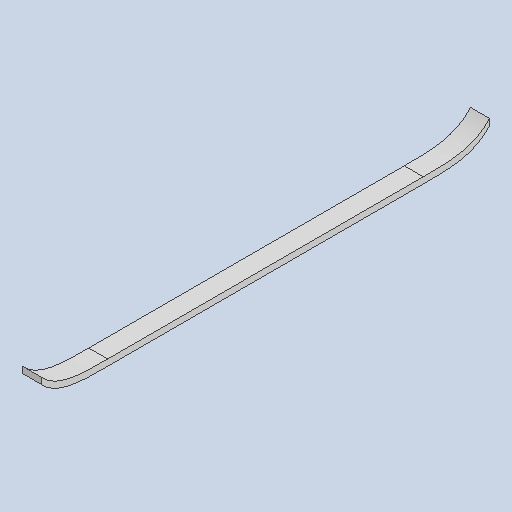
# Autodesk Inventor part: Landing_Skid
Saved by Autodesk Inventor 2027.1 (Build 311270010, 270A)
## iProperties
Created: 2026-09-09
Part Number: Landing_Skid
Material: Generic
Document SubType Name: Modeling
Designer: PWYNNE
Density: 1 g/cm^3
Appearance: Default
Author: PWYNNE
Autodesk Inventor part; units mm, degrees
ref_plane "YZ Plane" through (0, 0, 0) normal (1, 0, 0) x (0, 1, 0)
sketch "Sketch2" plane through (0, 0, 0) normal (1, 0, 0) x (0, 1, 0)
  line L0 (0, 0) -> (10, 0)
  line L1 (10, 0) -> (10, -500)
  line L2 (10, -500) -> (0, -500)
  line L3 (0, -500) -> (0, 0)
  line L4 (0, -500) -> (0, -541.4282) construction
  line L5 (0, -541.4282) -> (0, -581.277) construction
  line L6 (0, -581.277) -> (27.5525, -604.9907) construction
  spline S0 degree 3 poles (0, -500) (0, -541.4282) (0, -581.277) (27.5525, -604.9907) knots 1 1 1 1 2 2 2 2
  line L7 (10, -500) -> (10, -541.4282) construction
  line L8 (10, -541.4282) -> (10, -581.277) construction
  line L9 (10, -581.277) -> (37.5525, -604.9907) construction
  spline S1 degree 3 poles (10, -500) (10, -541.4282) (10, -581.277) (37.5525, -604.9907) knots 1 1 1 1 2 2 2 2
  line L10 (37.5525, -604.9907) -> (27.5525, -604.9907)
  line L11 (0, -250) -> (10, -250)
  line L12 (0, 0) -> (0, 41.4282) construction
  line L13 (0, 41.4282) -> (0, 81.277) construction
  line L14 (0, 81.277) -> (27.5525, 104.9907) construction
  spline S2 degree 3 poles (0, 0) (0, 41.4282) (0, 81.277) (27.5525, 104.9907) knots 1 1 1 1 2 2 2 2
  spline S3 degree 3 poles (10, 0) (10, 41.4282) (10, 81.277) (37.5525, 104.9907) knots 1 1 1 1 2 2 2 2
  line L15 (10, 0) -> (10, 41.4282) construction
  line L16 (10, 41.4282) -> (10, 81.277) construction
  line L17 (10, 81.277) -> (37.5525, 104.9907) construction
  line L18 (37.5525, 104.9907) -> (27.5525, 104.9907)
  dimension "d0" = 500
  dimension "d1" = 10
  constraints: 14 end point, 7 symmetric about line, 4 vertical, 3 horizontal, 2 midpoint, 2 parallel, 1 perpendicular, 12 other
  measures "d0" distance of L0.end L1.end
  measures "d1" distance of L1.end L2.end
extrude "Extrusion1" add sketch "Sketch2" along normal blind 30
ref_plane "Work Plane1" through (30, 10, 0) normal (0, 0, 1) x (-1, 0, 0)
ref_plane "Work Plane2" through (30, 0, -500) normal (0, 0, 1) x (0, 1, 0)
body "Solid1"
